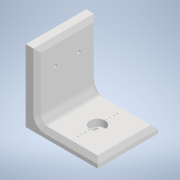
# Autodesk Inventor part: ToiletBowl2.0
Saved by Autodesk Inventor 2020 (Build 240168000, 168)
## iProperties
Created: 2020-04-13
Part Number: ToiletBowl2.0
Material: Generic
Document SubType Name: Modeling
Designer: varun
Density: 1 g/cm^3
Appearance: Default
Author: varun
Autodesk Inventor part; units mm, degrees
ref_plane "YZ Plane" through (0, 0, 0) normal (1, 0, 0) x (0, 1, 0)
ref_plane "XZ Plane" through (0, 0, 0) normal (0, 1, 0) x (-1, 0, 0)
ref_plane "XY Plane" through (0, 0, 0) normal (0, 0, 1) x (1, 0, 0)
sketch "Sketch1" plane through (0, 0, 0) normal (0, 1, 0) x (-1, 0, 0)
  line L0 (-25.4, 25.4) -> (25.4, 25.4)
  line L1 (25.4, 25.4) -> (25.4, -25.4)
  line L2 (25.4, -25.4) -> (-25.4, -25.4)
  line L3 (-25.4, -25.4) -> (-25.4, 25.4)
  line L4 (-25.4, 25.4) -> (25.4, -25.4) construction
  line L5 (25.4, 25.4) -> (-25.4, -25.4) construction
  point P0 (0, 0)
  dimension "d0" = 50.8
  dimension "d1" = 50.8
  constraints: 12 end point, 2 midpoint, 2 parallel, 1 horizontal, 1 perpendicular
  measures "d0" distance of L1.end L2.end
  measures "d1" distance of L0.end L1.end
extrude "Extrusion1" add sketch "Sketch1" along normal blind 12.7
sketch "Sketch2" plane through (-25.4, 0, -25.4) normal (-1, 0, 0) x (0, 0, 1)
  line L0 (0, 0) -> (50.8, 0) projected
  line L1 (50.8, 0) -> (50.8, 12.7) projected
  line L2 (0, 12.7) -> (50.8, 12.7) projected
  line L3 (0, 0) -> (0, 12.7) projected
  point P0 (25.4, 0)
extrude "Extrusion2" add sketch "Sketch2" along normal blind 12.7
sketch "Sketch3" plane through (0, 12.7, 0) normal (0, 1, 0) x (1, 0, 0)
  line L0 (25.4, 25.4) -> (-38.1, 25.4) projected
  line L1 (25.4, -25.4) -> (-38.1, -25.4) projected
  line L2 (-38.1, 25.4) -> (-25.4, 25.4)
  line L3 (-25.4, 25.4) -> (-25.4, -25.4)
  line L4 (-25.4, -25.4) -> (-38.1, -25.4)
  line L5 (-38.1, -25.4) -> (-38.1, 25.4)
  point P0 (0, 0)
  point P1 (-38.1, -25.4)
  dimension "d6" = 12.7
  constraints: 8 end point, 2 parallel, 1 horizontal, 1 perpendicular, 1 point on line
  measures "d6" distance of L3.end L4.end
extrude "Extrusion3" add sketch "Sketch3" along normal blind 50.8
sketch "Sketch4" plane through (0, 12.7, 0) normal (0, 1, 0) x (1, 0, 0)
  line L0 (22.225, 22.225) -> (-22.225, 22.225)
  line L1 (-22.225, 22.225) -> (-22.225, -22.225)
  line L2 (-22.225, -22.225) -> (22.225, -22.225)
  line L3 (22.225, -22.225) -> (22.225, 22.225)
  line L4 (22.225, 22.225) -> (-22.225, -22.225) construction
  line L5 (-22.225, 22.225) -> (22.225, -22.225) construction
  point P0 (0, 0)
  dimension "d9" = 44.45
  dimension "d10" = 44.45
  constraints: 12 end point, 2 midpoint, 2 parallel, 1 horizontal, 1 perpendicular
  measures "d9" distance of L2.end L1.end
  measures "d10" distance of L1.end L0.end
extrude "Extrusion4" cut sketch "Sketch4" against normal blind 7.62
sketch "Sketch5" plane through (0, 5.08, 0) normal (0, 1, 0) x (1, 0, 0)
  point P0 (0, 0)
sketch "Sketch6" plane through (0, 0, 0) normal (0, -1, 0) x (1, 0, 0)
  line L0 (-4.8916, 4.049) -> (-2.6097, 16.9902)
  line L1 (-4.8916, -4.049) -> (-2.6097, -16.9902)
  line L2 (2.6097, -16.9902) -> (4.8916, -4.049)
  line L3 (2.6097, 16.9902) -> (4.8916, 4.049)
  arc A0 (-4.8916, 4.049) -> (-4.8916, -4.049) centre (0, 0) ccw
  arc A1 (4.8916, -4.049) -> (4.8916, 4.049) centre (0, 0) ccw
  arc A2 (2.6097, 16.9902) -> (-2.6097, 16.9902) centre (0, 16.53) ccw
  arc A3 (-2.6097, -16.9902) -> (2.6097, -16.9902) centre (0, -16.53) ccw
  circle A4 centre (0, 0) radius 1.4
  circle A5 centre (0, 7.53) radius 0.5
  circle A6 centre (0, 10.53) radius 0.5
  circle A7 centre (0, 13.53) radius 0.5
  circle A8 centre (0, 16.53) radius 0.5
  circle A9 centre (0, -16.53) radius 0.5
  circle A10 centre (0, -13.53) radius 0.5
  circle A11 centre (0, -10.53) radius 0.5
  circle A12 centre (0, -7.53) radius 0.5
  point P0 (0, 0)
  constraints: 13 centre point, 8 end point, 8 point on circle, 3 coincident
extrude "Extrusion5" cut sketch "Sketch6" against normal up to surface (5.08 mm away) contours A5 | A6 | A7 | A8 | A10 | A11 | A12
sketch "Sketch7" plane through (0, 0, 0) normal (0, -1, 0) x (1, 0, 0)
  line L0 (-4.8916, 4.049) -> (-2.6097, 16.9902)
  line L1 (-4.8916, -4.049) -> (-2.6097, -16.9902)
  line L2 (2.6097, -16.9902) -> (4.8916, -4.049)
  line L3 (2.6097, 16.9902) -> (4.8916, 4.049)
  arc A0 (-4.8916, 4.049) -> (-4.8916, -4.049) centre (0, 0) ccw
  arc A1 (4.8916, -4.049) -> (4.8916, 4.049) centre (0, 0) ccw
  arc A2 (2.6097, 16.9902) -> (-2.6097, 16.9902) centre (0, 16.53) ccw
  arc A3 (-2.6097, -16.9902) -> (2.6097, -16.9902) centre (0, -16.53) ccw
  circle A4 centre (0, 0) radius 1.4
  circle A5 centre (0, 7.53) radius 0.5
  circle A6 centre (0, 10.53) radius 0.5
  circle A7 centre (0, 13.53) radius 0.5
  circle A8 centre (0, 16.53) radius 0.5
  circle A9 centre (0, -16.53) radius 0.5
  circle A10 centre (0, -13.53) radius 0.5
  circle A11 centre (0, -10.53) radius 0.5
  circle A12 centre (0, -7.53) radius 0.5
  point P0 (-4.8916, 4.049)
  point P1 (-2.6097, 16.9902)
  constraints: 13 centre point, 8 end point, 8 point on circle, 3 coincident
extrude "Extrusion6" cut sketch "Sketch7" against normal blind 3.81
sketch "Sketch8" plane through (0, 0, 0) normal (0, -1, 0) x (1, 0, 0)
  circle A0 centre (0, 0) radius 6.35
  point P0 (4.8916, 4.049)
  constraints: 1 coincident, 3 other
extrude "Extrusion7" cut sketch "Sketch8" against normal up to surface (5.08 mm away)
sketch "Sketch10" plane through (0, 5.08, 0) normal (0, 1, 0) x (1, 0, 0)
  circle A0 centre (0, 0) radius 6.35 projected
  circle A1 centre (0, -10.53) radius 0.5 projected
  circle A2 centre (0, -16.53) radius 0.5 projected
  circle A3 centre (0, 7.53) radius 0.5 projected
  circle A4 centre (0, 10.53) radius 0.5 projected
  circle A5 centre (0, -13.53) radius 0.5 projected
  circle A6 centre (0, -7.53) radius 0.5 projected
  circle A7 centre (0, 13.53) radius 0.5 projected
  line L0 (22.225, 22.225) -> (22.225, -22.225) projected
  line L1 (-22.225, 22.225) -> (22.225, 22.225) projected
  line L2 (-22.225, -22.225) -> (-22.225, 22.225) projected
  line L3 (22.225, -22.225) -> (-22.225, -22.225) projected
extrude "Extrusion9" add sketch "Sketch10" along normal up to surface (7.62 mm away)
sketch "Sketch11" plane through (0, 12.7, 0) normal (0, 1, 0) x (1, 0, 0)
  line L0 (25.4, -25.4) -> (-25.4, -25.4) projected
  line L1 (25.4, -25.4) -> (25.4, 25.4) projected
  line L2 (25.4, 25.4) -> (-25.4, 25.4) projected
  circle A0 centre (0, 0) radius 6.35 projected
  circle A1 centre (0, -10.53) radius 0.5 projected
  circle A2 centre (0, -16.53) radius 0.5 projected
  circle A3 centre (0, 7.53) radius 0.5 projected
  circle A4 centre (0, 10.53) radius 0.5 projected
  circle A5 centre (0, -13.53) radius 0.5 projected
  circle A6 centre (0, -7.53) radius 0.5 projected
  circle A7 centre (0, 13.53) radius 0.5 projected
  line L3 (-25.4, 25.4) -> (-25.4, -25.4) projected
extrude "Extrusion10" cut sketch "Sketch11" against normal blind 3.175
sketch "Sketch12" plane through (0, 0, -16.53) normal (0, -1, 0) x (1, 0, 0)
  circle A0 centre (0, 0) radius 0.5 projected
  point P0 (0, 16.53)
extrude "Extrusion11" cut sketch "Sketch12" against normal up to surface (9.525 mm away)
sketch "Sketch13" plane through (0, 0, 0) normal (0, -1, 0) x (1, 0, 0)
  arc A0 (-2.6097, -16.9902) -> (2.6097, -16.9902) centre (0, -16.53) ccw projected
  line L0 (-2.6097, -16.9902) -> (-4.8916, -4.049) projected
  arc A1 (-4.8916, 4.049) -> (-4.8916, -4.049) centre (0, 0) ccw projected
  line L1 (-4.8916, 4.049) -> (-2.6097, 16.9902) projected
  arc A2 (2.6097, 16.9902) -> (-2.6097, 16.9902) centre (0, 16.53) ccw projected
  line L2 (2.6097, 16.9902) -> (4.8916, 4.049) projected
  arc A3 (4.8916, -4.049) -> (4.8916, 4.049) centre (0, 0) ccw projected
  line L3 (4.8916, -4.049) -> (2.6097, -16.9902) projected
  line L4 (-38.1, 25.4) -> (25.4, 25.4) projected
  line L5 (-38.1, -25.4) -> (-38.1, 25.4) projected
  line L6 (25.4, -25.4) -> (-38.1, -25.4) projected
  line L7 (25.4, 25.4) -> (25.4, -25.4) projected
  arc A4 (-2.3037, -16.9362) -> (2.3037, -16.9362) centre (0, -16.53) ccw
  line L8 (-2.3037, -16.9362) -> (-4.6, -3.9131)
  arc A5 (-4.6, 3.9131) -> (-4.6, -3.9131) centre (0, 0) ccw
  line L9 (-4.6, 3.9131) -> (-2.3037, 16.9362)
  arc A6 (2.3037, 16.9362) -> (-2.3037, 16.9362) centre (0, 16.53) ccw
  line L10 (2.3037, 16.9362) -> (4.6, 3.9131)
  arc A7 (4.6, -3.9131) -> (4.6, 3.9131) centre (0, 0) ccw
  line L11 (4.6, -3.9131) -> (2.3037, -16.9362)
  constraints: 8 end point, 8 point on circle, 4 centre point, 7 other
extrude "Extrusion12" add sketch "Sketch13" against normal blind 3.65 contours L8 A5 L9 A6 L10 A7 L11 A4
sketch "Sketch14" plane through (0, 0, 0) normal (0, -1, 0) x (1, 0, 0)
  line L0 (-2.3037, 16.9362) -> (-4.6, 3.9131) projected
  arc A0 (-4.6, 3.9131) -> (-4.6, -3.9131) centre (0, 0) ccw projected
  line L1 (-4.6, -3.9131) -> (-2.3037, -16.9362) projected
  arc A1 (-2.3037, -16.9362) -> (2.3037, -16.9362) centre (0, -16.53) ccw projected
  line L2 (2.3037, -16.9362) -> (4.6, -3.9131) projected
  arc A2 (4.6, -3.9131) -> (4.6, 3.9131) centre (0, 0) ccw projected
  line L3 (4.6, 3.9131) -> (2.3037, 16.9362) projected
  arc A3 (2.3037, 16.9362) -> (-2.3037, 16.9362) centre (0, 16.53) ccw projected
  arc A4 (-4.0301, 3.6399) -> (-4.0301, -3.6399) centre (0, 0) ccw
  line L4 (-4.0301, 3.6399) -> (-1.7042, 16.8305)
  arc A5 (1.7042, 16.8305) -> (-1.7042, 16.8305) centre (0, 16.53) ccw
  line L5 (1.7042, 16.8305) -> (4.0301, 3.6399)
  arc A6 (4.0301, -3.6399) -> (4.0301, 3.6399) centre (0, 0) ccw
  line L6 (4.0301, -3.6399) -> (1.7042, -16.8305)
  arc A7 (-1.7042, -16.8305) -> (1.7042, -16.8305) centre (0, -16.53) ccw
  line L7 (-1.7042, -16.8305) -> (-4.0301, -3.6399)
  line L8 (-4.0301, -3.6399) -> (-2.8671, -3.6399)
  line L9 (-2.8671, -3.6399) -> (-4.0301, 3.6399)
  line L10 (-2.8671, -3.6399) -> (-2.8671, 3.6399)
  line L11 (-2.8671, 3.6399) -> (-4.0301, 3.6399)
  point P0 (-4.0301, -3.6399)
  constraints: 16 end point, 8 point on circle, 4 centre point, 2 perpendicular, 1 horizontal, 7 other
extrude "Extrusion13" cut sketch "Sketch14" against normal blind 3.65 contours L9 L8 A4 | L11 L10 L9
fillet "Fillet3" radius 6.35 1 edges at (-25.4, 9.525, 0)
chamfer "Chamfer3" distance 3.175 angle 45 14 edges at (-6.35, 0, -25.4) (25.4, 0, 0) (-6.35, 0, 25.4) (-38.1, 31.75, 25.4) (-38.1, 31.75, -25.4) (-38.1, 63.5, 0) (-25.4, 39.6875, 25.4) (-23.5401, 11.3849, 25.4) (3.175, 9.525, 25.4) (-25.4, 63.5, 0) (-25.4, 39.6875, -25.4) (-23.5401, 11.3849, -25.4) (3.175, 9.525, -25.4) (25.4, 9.525, 0)
chamfer "Chamfer4" distance 3.175 angle 45 1 edges at (-38.1, 0, 0)
sketch "Sketch15" plane through (-25.4, 15.875, -22.225) normal (1, 0, 0) x (0, 0, -1)
  line L0 (-1.725, 37.125) -> (-1.725, 17.125) projected
  arc A0 (-1.725, 37.125) -> (-5.725, 41.125) centre (-5.725, 37.125) ccw projected
  line L1 (-5.725, 41.125) -> (-38.725, 41.125) projected
  arc A1 (-38.725, 41.125) -> (-42.725, 37.125) centre (-38.725, 37.125) ccw projected
  line L2 (-42.725, 37.125) -> (-42.725, 17.125) projected
  line L3 (-1.725, 17.125) -> (-42.725, 17.125) projected
  circle A2 centre (-32.225, 28.995) radius 1.25 projected
  circle A3 centre (-12.225, 28.995) radius 1.25 projected
  circle A4 centre (-12.225, 28.995) radius 1.25
  circle A5 centre (-32.225, 28.995) radius 1.25
  point P0 (-22.225, -15.875)
  constraints: 2 centre point, 2 coincident, 2 concentric
extrude "Extrusion14" cut sketch "Sketch15" against normal up to surface (12.7 mm away) contours A2 | A3
body "Solid1"
